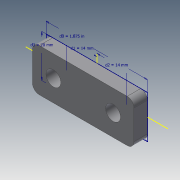
# Autodesk Inventor part: FLUGGER HINGE SPACER
Saved by Autodesk Inventor 2020.3 (Build 243373000, 373)
## iProperties
RuleStatus: InUse
AfterDocSave0: file://Part Number Cleaner
Created: 2020-01-10
Material: Generic
Vendor: HHMI: JRC - ID&F
Document SubType Name: Modeling
Designer: arnoldj
Density: 1 g/cm^3
Appearance: Default
DESIGN DEPARTMENT: HHMI: JRC - ID&F
ALTERED ITEM PART NUMBER: N/A
ALTERED ITEM VENDOR: N/A
ALTERED ITEM DESCRIPTION: N/A
Author: arnoldj
Revision Number: 0
Autodesk Inventor part; units mm, degrees
ref_plane "YZ Plane" through (0, 0, 0) normal (1, 0, 0) x (0, 1, 0)
ref_plane "XZ Plane" through (0, 0, 0) normal (0, 1, 0) x (-1, 0, 0)
ref_plane "XY Plane" through (0, 0, 0) normal (0, 0, 1) x (1, 0, 0)
sketch "Sketch1" plane through (0, 0, 0) normal (0, 0, 1) x (1, 0, 0)
  line L0 (0, 14) -> (0, -14) projected
  line L1 (-33.3375, 0) -> (33.3375, 0) projected
  line L2 (23.8125, -10) -> (-23.8125, -10)
  line L3 (-23.8125, -10) -> (-23.8125, 10)
  line L4 (-23.8125, 10) -> (23.8125, 10)
  line L5 (23.8125, 10) -> (23.8125, -10)
  line L6 (23.8125, -10) -> (-23.8125, 10) construction
  line L7 (-23.8125, -10) -> (23.8125, 10) construction
  point P0 (0, 0)
  point P1 (-14, 0)
  point P2 (14, 0)
  dimension "d0" = 47.625
  dimension "d1" = 14
  dimension "d2" = 14
  dimension "d3" = 20
  constraints: 12 end point, 2 equal length, 2 midpoint, 2 point on line, 1 parallel, 1 vertical
  measures "d0" distance of L3.end L4.end
  measures "d1" distance from line of L0 point (-14, 0)
  measures "d2" distance from line of L0 point (14, 0)
  measures "d3" distance of L2.end L3.end
extrude "Extrusion1" add sketch "Sketch1" along normal blind 6.35
hole "Hole1" at (-14, 0, 0) at (14, 0, 0) direction (0, 0, 1) diameter 6.985 end through all
fillet "Fillet1" radius 3.175 4 edges at (23.8125, 10, 3.175) (23.8125, -10, 3.175) (-23.8125, -10, 3.175) (-23.8125, 10, 3.175)
body "Solid1"
